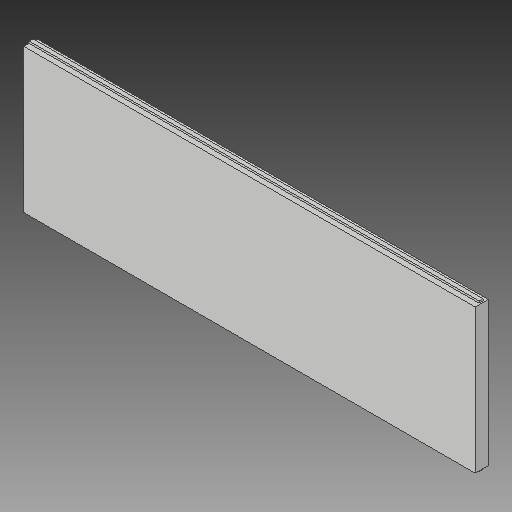
# Autodesk Inventor part: Bovenkant
Saved by Autodesk Inventor 2018.3 (Build 223284000, 284)
## iProperties
Created: 2020-11-10
Part Number: Bovenkant
Material: Generic
Document SubType Name: Modeling
Designer: daanv
Density: 1 g/cm^3
Appearance: Default
Author: daanv
## iProperties of the stored document Bovenkant_3DPrint.ipt
Created: 2020-11-17
Part Number: Bovenkant_3DPrint
Material: Generic
Document SubType Name: Modeling
Designer: daanv
Density: 1 g/cm^3
Appearance: Default
Author: daanv
Autodesk Inventor part; units mm, degrees
ref_plane "YZ Plane" through (0, 0, 0) normal (1, 0, 0) x (0, 1, 0)
ref_plane "XZ Plane" through (0, 0, 0) normal (0, 1, 0) x (-1, 0, 0)
ref_plane "XY Plane" through (0, 0, 0) normal (0, 0, 1) x (1, 0, 0)
sketch "Sketch1" plane through (0, 0, 0) normal (0, 0, 1) x (1, 0, 0)
  line L0 (0, 0) -> (34.5, 0)
  line L1 (34.5, 0) -> (34.5, 11)
  line L2 (34.5, 11) -> (0, 11)
  line L3 (0, 11) -> (0, 0)
  dimension "d0" = 34.5
  dimension "d1" = 11
  constraints: 8 end point, 2 parallel, 1 horizontal, 1 perpendicular
  measures "d0" distance of L2.end L1.end
  measures "d1" distance of L1.end L0.end
extrude "Extrusion1" add sketch "Sketch1" along normal blind 1
sketch "Sketch2" plane through (0, 0, 0) normal (-1, 0, 0) x (0, 0, 1)
  line L0 (1, 11) -> (1, 0) projected
  line L1 (0, 11) -> (1, 11) projected
  line L2 (0.6, 11) -> (0.3, 11)
  line L3 (0.3, 11) -> (0.3, 11.15)
  line L4 (0.3, 11.15) -> (0.6, 11.15)
  line L5 (0.6, 11.15) -> (0.6, 11)
  line L6 (0, 0) -> (1, 0) projected
  line L7 (0.6, 0) -> (0.3, 0)
  line L8 (0.3, 0) -> (0.3, -0.15)
  line L9 (0.3, -0.15) -> (0.6, -0.15)
  line L10 (0.6, -0.15) -> (0.6, 0)
  dimension "d4" = 0.3
  dimension "d5" = 0.15
  dimension "d6" = 0.4
  dimension "d7" = 0.15
  constraints: 16 end point, 4 parallel, 2 horizontal, 2 perpendicular, 2 point on line
  measures "d4" distance of L3.end L4.end
  measures "d5" distance of L2.end L3.end
  measures "d6" distance between parallel lines of L0 L5
  measures "d7" distance of L8.end L7.end
extrude "Extrusion2" add sketch "Sketch2" against normal blind 34.5
sketch "Sketch3" plane through (0, -0.15, 0.3) normal (0, -1, 0) x (1, 0, 0)
  line L0 (0, 0.3) -> (34.5, 0.3) projected
  line L1 (34.5, 0) -> (0, 0) projected
  line L2 (34.5, 0.3) -> (34.4, 0.3)
  line L3 (34.4, 0.3) -> (34.4, 0)
  line L4 (34.4, 0) -> (34.5, 0)
  line L5 (34.5, 0) -> (34.5, 0.3)
  point P0 (0, -0.3)
  dimension "d10" = 0.1
  constraints: 8 end point, 2 parallel, 1 horizontal, 1 perpendicular, 1 point on line
  measures "d10" distance of L4.end L3.end
extrude "Extrusion3" cut sketch "Sketch3" against normal blind 0.15
sketch "Sketch4" plane through (0, 11.15, 0.6) normal (0, 1, 0) x (1, 0, 0)
  line L0 (34.4, 0.3) -> (0, 0.3) projected
  line L1 (34.5, 0) -> (34.4, 0)
  line L2 (34.4, 0) -> (34.4, 0.3)
  line L3 (34.4, 0.3) -> (34.5, 0.3)
  line L4 (34.5, 0.3) -> (34.5, 0)
  point P0 (0, 0.6)
  dimension "d13" = 0.1
  constraints: 8 end point, 2 parallel, 1 horizontal, 1 perpendicular
  measures "d13" distance of L0.start L3.end
extrude "Extrusion4" cut sketch "Sketch4" against normal blind 0.15
body "Solid1"
